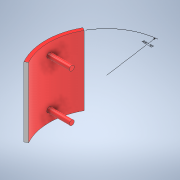
# Autodesk Inventor part: airframe
Saved by Autodesk Inventor 2022 (Build 260153000, 153)
## iProperties
Created: 2021-07-21
Part Number: airframe
Material: Generic
Document SubType Name: Modeling
Designer: WASHINGTON
Density: 1 g/cm^3
Appearance: Default
Author: WASHINGTON
Autodesk Inventor part; units mm, degrees
ref_plane "YZ Plane" through (0, 0, 0) normal (1, 0, 0) x (0, 1, 0)
ref_plane "XZ Plane" through (0, 0, 0) normal (0, 1, 0) x (-1, 0, 0)
ref_plane "XY Plane" through (0, 0, 0) normal (0, 0, 1) x (1, 0, 0)
sketch "Sketch1" plane through (0, 0, 0) normal (0, 1, 0) x (-1, 0, 0)
  arc A0 (-87.5, 0) -> (0, 87.5) centre (0, 0) ccw
  arc A1 (-82.5, 0) -> (0, 82.5) centre (0, 0) ccw
  line L0 (0, 87.5) -> (0, 82.5)
  line L1 (-82.5, 0) -> (-87.5, 0)
  dimension "d0" = 165
  dimension "d1" = 175
  dimension "d7" = 0
  dimension "d8" = 0
  constraints: 4 end point, 4 point on circle, 2 centre point, 2 coincident, 1 perpendicular, 1 vertical
  measures "d0" diameter of A1
  measures "d1" diameter of A0
  measures "d7" distance from line of point (0, 0) L0
  measures "d8" distance from line of point (0, 0) L1
extrude "Extrusion1" add sketch "Sketch1" along normal mid plane 100
sketch "Sketch5" plane through (0, 0, 0) normal (1, 0, 0) x (0, 1, 0)
  line L0 (-50, 0) -> (50, 0) projected
  circle A0 centre (34, 0) radius 3.5
  circle A1 centre (-34, 0) radius 3.5
  point P0 (0, 0)
  dimension "d22" = 7
  dimension "d23" = 7
  dimension "d24" = 68
  dimension "d25" = 34
  constraints: 2 centre point, 2 point on line
  measures "d22" diameter of A0
  measures "d23" diameter of A1
  measures "d24" distance of A1.centre A0.centre
  measures "d25" distance of point (0, 0) A0.centre
extrude "Extrusion4" add sketch "Sketch5" against normal up to next
sketch "Sketch6" plane through (0, 34, 0) normal (1, 0, 0) x (0, 0, -1)
  circle A0 centre (0, 0) radius 3.5
  line L0 (0, -84) -> (0, 16) projected
  circle A1 centre (0, -68.0281) radius 3.5281
  point P0 (0, -34)
  constraints: 2 centre point, 1 point on line
extrude "Extrusion5" cut sketch "Sketch6" against normal blind 50
sketch "Sketch7" plane through (0, 50, 0) normal (0, 1, 0) x (1, 0, 0)
  arc A0 (87.5, 0) -> (0, -87.5) centre (0, 0) ccw construction
  arc A1 (82.5, 0) -> (0, -82.5) centre (0, 0) ccw construction
  arc A2 (-87.5, 0) -> (-76.5573, -42.3702) centre (0, 0) ccw
  arc A3 (-82.5, 0) -> (-72.2264, -39.8698) centre (0, 0) ccw
  line L0 (-72.2264, -39.8698) -> (-76.5573, -42.3702)
  line L1 (0, 0) -> (-87.5, 0) construction
  arc A4 (0, 87.5) -> (87.5, 0) centre (0, 0) ccw construction
  arc A5 (0, 82.5) -> (82.5, 0) centre (0, 0) ccw construction
  arc A6 (-76.5573, 42.3702) -> (-87.5, 0) centre (0, 0) ccw
  arc A7 (-72.2264, 39.8698) -> (-82.5, 0) centre (0, 0) ccw
  line L2 (-72.2264, 39.8698) -> (-76.5573, 42.3702)
  arc A8 (82.5, 0) -> (-72.2264, 39.8698) centre (0, 0) ccw
  arc A9 (87.5, 0) -> (-76.5573, 42.3702) centre (0, 0) ccw
  arc A10 (-76.5573, -42.3702) -> (0, -87.5) centre (0, 0) ccw
  arc A11 (-72.2264, -39.8698) -> (0, -82.5) centre (0, 0) ccw
  line L3 (-156.1445, -133.794) -> (99.266, -133.794)
  line L4 (99.266, -133.794) -> (99.266, 159.7464)
  line L5 (99.266, 159.7464) -> (-156.1445, 159.7464)
  line L6 (-156.1445, 159.7464) -> (-156.1445, -133.794)
  circle A12 centre (0, 0) radius 82.5
  point P0 (0, -82.5)
  dimension "d30" = 30
  dimension "d31" = 45.3349
  dimension "d32" = 0
  dimension "d33" = 255.4104
  dimension "d34" = 293.5404
  dimension "d35" = 159.7464
  dimension "d36" = 11.766
  constraints: 26 point on circle, 14 end point, 10 centre point, 9 coincident, 4 symmetric about line, 2 concentric, 2 horizontal, 2 parallel, 1 perpendicular, 7 other
  measures "d30" angle of L2 L1
  measures "d31" distance from line of A0.start L2
  measures "d32" distance from line of A3.start L1
  measures "d33" distance between parallel lines of L4 L6
  measures "d34" distance between parallel lines of L3 L5
  measures "d35" distance between parallel lines of L5 L1
  measures "d36" distance from line of A0.start L4
extrude "Extrusion6" cut sketch "Sketch7" against normal up to next
sketch "Sketch3" plane through (0, 0, 0) normal (1, 0, 0) x (0, 1, 0)
  circle A0 centre (0, 34) radius 3.5
  circle A1 centre (0, -34) radius 3.5
  circle A2 centre (0, 34) radius 3.5
  circle A3 centre (0, -34) radius 3.5
  point P0 (0, 0)
  dimension "d9" = 7
  dimension "d10" = 7
  dimension "d11" = 68
  dimension "d12" = 34
  dimension "d13" = 34
  constraints: 4 centre point, 2 coincident, 2 concentric
  measures "d9" diameter of A0
  measures "d10" diameter of A1
  measures "d11" distance of A1.centre A0.centre
  measures "d12" distance of point (0, 0) A0.centre
  measures "d13" distance of point (0, 0) A1.centre
sketch "Sketch4" plane through (0, 0, 34) normal (1, 0, 0) x (0, 0, -1)
  circle A0 centre (0, 0) radius 3.5
  circle A1 centre (68, 0) radius 3.5 projected
  circle A2 centre (68, 0) radius 3.5
  point P0 (34, 0)
  constraints: 2 centre point, 1 coincident
equation "\"d26\" = d23"
body "Solid1"
